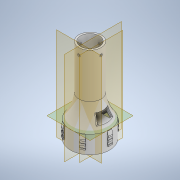
# Autodesk Inventor part: Tube_1
Saved by Autodesk Inventor 2022.3 (Build 263350000, 350)
## iProperties
Created: 2023-03-28
Part Number: Tube_1
Material: Generic
Document SubType Name: Modeling
Designer: Manuel Hueso Béjar
Density: 1 g/cm^3
Appearance: Default
Author: Manuel Hueso Béjar
Autodesk Inventor part; units mm, degrees
ref_plane "XZ Plane" through (0, 0, 0) normal (0, 1, 0) x (-1, 0, 0)
sketch "Sketch1" plane through (0, 0, 0) normal (0, 1, 0) x (-1, 0, 0)
  circle A0 centre (0, 0) radius 40
  circle A1 centre (0, 0) radius 44
  dimension "d0" = 80
  dimension "d1" = 4
  constraints: 2 centre point, 1 coincident
  measures "d0" diameter of A0
  measures "d1" radial gap between concentric circles of A0 A1
extrude "Extrusion1" add sketch "Sketch1" along normal blind 40
sketch "Sketch2" plane through (0, 0, 0) normal (0, 0, 1) x (1, 0, 0)
  line L0 (44, 40) -> (-44, 40) projected
  line L1 (-44, 40) -> (44, 40)
  line L2 (44, 40) -> (44, 90)
  line L3 (44, 90) -> (-44, 90)
  line L4 (-44, 90) -> (-44, 40)
  line L5 (25, 40) -> (-25, 40)
  arc A0 (-44, 40) -> (-25, 90) centre (-124.5733, 99.2279) ccw
  line L6 (-25, 90) -> (0, 90)
  line L7 (0, 90) -> (0, 190)
  line L8 (0, 190) -> (-25, 190)
  line L9 (-25, 190) -> (-25, 90)
  line L10 (0, 90) -> (0, 40)
  line L11 (0, 40) -> (-44, 40)
  line L12 (-25, 190) -> (-21, 190)
  line L13 (-21, 190) -> (-21, 90)
  line L14 (-21, 90) -> (-25, 90)
  line L15 (-25, 90) -> (-25, 190)
  line L16 (-40, 40) -> (40, 40) projected
  arc A1 (-40, 40) -> (-21, 90) centre (-120.5733, 99.2279) ccw
  line L17 (-21, 90) -> (-41, 90)
  line L18 (-41, 90) -> (-41, 70)
  line L19 (-41, 70) -> (-21, 70)
  line L20 (-21, 70) -> (-21, 90)
  line L21 (-44, 40) -> (-29, 40)
  line L22 (-29, 40) -> (-29, 50)
  line L23 (-29, 50) -> (-44, 50)
  line L24 (-44, 50) -> (-44, 40)
  arc A2 (-40.8057, 40.5923) -> (-21.9957, 90.0923) centre (-120.5733, 99.2279) ccw
  line L25 (-24.94, 70) -> (-29.94, 70)
  line L26 (-29.94, 70) -> (-29.94, 68)
  line L27 (-29.94, 68) -> (-24.94, 68)
  line L28 (-24.94, 68) -> (-24.94, 70)
  line L29 (-37.5296, 50) -> (-32.5296, 50)
  line L30 (-32.5296, 50) -> (-32.5296, 51)
  line L31 (-32.5296, 51) -> (-37.5296, 51)
  line L32 (-37.5296, 51) -> (-37.5296, 50)
  point P0 (0, 0)
  point P1 (0, 90)
  point P2 (-25, 90)
  point P3 (-28.94, 70)
  point P4 (-37.5296, 50)
  point P5 (-33.5296, 50)
  point P6 (-25.9862, 70)
  point P7 (-34.6803, 50)
  point P8 (-25.5743, 68)
  point P9 (-26.6275, 68)
  dimension "d4" = 88
  dimension "d5" = 50
  dimension "d8" = 100
  dimension "d9" = 25
  dimension "d10" = 100
  dimension "d11" = 4
  dimension "d12" = 100
  dimension "d79" = 0
  dimension "d196" = 20
  dimension "d197" = 20
  dimension "d198" = 15
  dimension "d199" = 10
  dimension "d205" = 1
  dimension "d206" = 5
  dimension "d207" = 2
  dimension "d208" = 5
  dimension "d209" = 1
  constraints: 62 end point, 14 parallel, 8 perpendicular, 8 point on circle, 7 horizontal, 3 centre point, 3 point on line, 2 midpoint
  measures "d4" distance of L3.end L2.end
  measures "d5" distance of L2.end L1.end
  measures "d8" radius of A0
  measures "d9" distance of L8.end L7.end
  measures "d10" distance of L7.end L6.end
  measures "d11" distance of L13.end L14.end
  measures "d12" radius of A1
  measures "d79" distance between parallel lines of L3 L6
  measures "d196" distance of L19.end L18.end
  measures "d197" distance of L18.end L17.end
  measures "d198" distance of L23.end L22.end
  measures "d199" distance of L22.end L21.end
  measures "d205" radial gap between concentric circles of A1 A2
  measures "d206" distance of L27.end L26.end
  measures "d207" distance of L26.end L25.end
  measures "d208" distance of L31.end L30.end
  measures "d209" distance of L30.end L29.end
revolve "Revolution1" add sketch "Sketch2" angle 360 about axis through (0, 90, 0) along (0, 1, 0) contours A1 L19 A2 L3 | L3 L9 L8 L13 | A2 L19 A0 L3 | A1 L27 A2 L19 | A2 L27 A0 L19 | A1 L31 A2 L27 | L0 A0 L23 A1 | A2 L31 A0 L27 | A1 L23 A2 L31 | A2 L23 A0 L31
ref_plane "Work Plane1" through (0, 45, 0) normal (0, -1, 0) x (1, 0, 0)
sketch "Sketch3" plane through (0, 45, 0) normal (0, -1, 0) x (1, 0, 0)
  line L0 (-2.5, -37.5) -> (2.5, -37.5)
  line L1 (2.5, -37.5) -> (2.5, 37.5)
  line L2 (2.5, 37.5) -> (-2.5, 37.5)
  line L3 (-2.5, 37.5) -> (-2.5, -37.5)
  circle A0 centre (0, 0) radius 44 projected
  line L4 (-2.5, -37.5) -> (2.5, 37.5) construction
  line L5 (2.5, -37.5) -> (-2.5, 37.5) construction
  line L6 (-37.5, -2.5) -> (37.5, -2.5)
  line L7 (37.5, -2.5) -> (37.5, 2.5)
  line L8 (37.5, 2.5) -> (-37.5, 2.5)
  line L9 (-37.5, 2.5) -> (-37.5, -2.5)
  line L10 (-37.5, -2.5) -> (37.5, 2.5) construction
  line L11 (37.5, -2.5) -> (-37.5, 2.5) construction
  circle A1 centre (0, 0) radius 7.5
  circle A2 centre (0, 0) radius 2.6
  circle A3 centre (0, 0) radius 6.6
  line L12 (37.5, 2.5) -> (2.5, 2.5)
  line L13 (2.5, 2.5) -> (2.5, 12.5)
  line L14 (2.5, 12.5) -> (37.5, 12.5)
  line L15 (37.5, 12.5) -> (37.5, 2.5)
  line L16 (-37.5, 2.5) -> (-2.5, 2.5)
  line L17 (-2.5, 2.5) -> (-2.5, 12.5)
  line L18 (-2.5, 12.5) -> (-37.5, 12.5)
  line L19 (-37.5, 12.5) -> (-37.5, 2.5)
  line L20 (37.5, -2.5) -> (-37.5, -2.5)
  line L21 (-37.5, -2.5) -> (-37.5, -12.5)
  line L22 (-37.5, -12.5) -> (37.5, -12.5)
  line L23 (37.5, -12.5) -> (37.5, -2.5)
  line L24 (-2.5, 37.5) -> (-12.5, 37.5)
  line L25 (-12.5, 37.5) -> (-12.5, -37.5)
  line L26 (-12.5, -37.5) -> (-2.5, -37.5)
  line L27 (-2.5, -37.5) -> (-2.5, 37.5)
  line L28 (2.5, 37.5) -> (12.5, 37.5)
  line L29 (12.5, 37.5) -> (12.5, -37.5)
  line L30 (12.5, -37.5) -> (2.5, -37.5)
  line L31 (2.5, -37.5) -> (2.5, 37.5)
  point P0 (7.0711, 2.5)
  point P1 (2.5, 7.0711)
  point P2 (-2.5, 7.0711)
  point P3 (-7.0711, 2.5)
  point P4 (-7.0711, -2.5)
  point P5 (-2.5, -7.0711)
  point P6 (2.5, -7.0711)
  point P7 (7.0711, -2.5)
  point P8 (2.5, 0.7141)
  point P9 (2.5, -0.7141)
  point P10 (12.5, 12.5)
  point P11 (-2.5, -0.7141)
  point P12 (-2.5, 0.7141)
  point P13 (-12.5, 12.5)
  point P14 (0.7141, -2.5)
  point P15 (-0.7141, -2.5)
  point P16 (-12.5, -12.5)
  point P17 (-2.5, -37.5)
  point P18 (12.5, -12.5)
  dimension "d15" = 5
  dimension "d16" = 75
  dimension "d17" = 75
  dimension "d18" = 5
  dimension "d19" = 15
  dimension "d20" = 5.2
  dimension "d165" = 4
  dimension "d181" = 10
  dimension "d182" = 10
  dimension "d202" = 10
  dimension "d203" = 10
  dimension "d204" = 10
  constraints: 64 end point, 14 parallel, 7 horizontal, 7 perpendicular, 4 midpoint, 3 centre point, 2 coincident, 2 point on line
  measures "d15" distance of L2.end L1.end
  measures "d16" distance of L1.end L0.end
  measures "d17" distance of L8.end L7.end
  measures "d18" distance of L7.end L6.end
  measures "d19" diameter of A1
  measures "d20" diameter of A2
  measures "d165" radial gap between concentric circles of A2 A3
  measures "d181" distance of L12.end L13.end
  measures "d182" distance of L17.end L16.end
  measures "d202" distance of L21.end L20.end
  measures "d203" distance of L26.end L25.end
  measures "d204" distance of L29.end L30.end
extrude "Extrusion2" add sketch "Sketch3" against normal blind 5 contours L3 L22 L1 L0 | L26 L25 L22 L3 | L1 L22 L29 L30 | L22 L25 L6 A1 L3 | L3 A1 L1 L22 | L1 A1 L6 L29 L22 | A1 L6 A3 L3 | L3 A3 L1 A1 | L22 L21 L6 L25 | L1 A3 L6 A1 | L29 L6 L23 L22 | A3 L6 L3 | L3 L6 A2 L1 A3 | A1 L8 A3 L6 | L6 L25 L8 A1 | L6 L9 L8 L25 | L1 L6 A3 | A1 L8 L29 L6 | L6 A3 L8 A1 | L29 L8 L7 L6 | L6 A3 L8 L3 A2 | L3 A2 L6 | A1 L3 A3 L8 | L8 L25 L18 L3 A1 | L8 L19 L18 L25 | L6 A2 L1 | L1 A2 L8 A3 L6 | L29 L14 L15 L8 | L8 A1 L1 L14 L29 | A2 L3 | L6 A2 | A3 L3 L8 | A1 L1 A3 L3 | L3 L2 L1 A1 | L25 L24 L3 L18 | L1 A2 | L8 A3 L1 A1 | L14 L1 L28 L29 | L3 L8 A2 | L3 A3 L1 L8 A2 | A2 L8 L1 | L8 L1 A3
sketch "Sketch18" plane through (0, 0, 0) normal (0, -1, 0) x (1, 0, 0)
  line L0 (-42, 5) -> (-46, 5)
  line L1 (-46, 5) -> (-46, -5)
  line L2 (-46, -5) -> (-42, -5)
  line L3 (-42, -5) -> (-42, 5)
  circle A0 centre (0, 0) radius 44 projected
  line L4 (-42, 5) -> (-46, -5) construction
  line L5 (-46, 5) -> (-42, -5) construction
  circle A1 centre (0, 0) radius 44
  point P0 (-44, 0)
  point P1 (-43.715, -5)
  point P2 (-43.715, 5)
  dimension "d106" = 4
  dimension "d107" = 10
  constraints: 12 end point, 2 midpoint, 2 parallel, 1 coincident, 1 horizontal, 1 horizontal alignment, 1 perpendicular, 4 other
  measures "d106" distance of L2.end L1.end
  measures "d107" distance of L1.end L0.end
extrude "Extrusion11" add sketch "Sketch18" against normal blind 30 contours A0 L2 L1 L0
sketch "Sketch19" plane through (-43.715, 0, -5) normal (0, 0, -1) x (-1, 0, 0)
  line L0 (0, 30) -> (2.285, 30) projected
  line L1 (0, 30) -> (2.285, 30)
  line L2 (2.285, 30) -> (2.285, 40)
  line L3 (2.285, 40) -> (0, 40)
  line L4 (0, 40) -> (0, 30)
  line L5 (0, 40) -> (2.285, 30)
  point P0 (-43.715, 0)
  dimension "d110" = 10
  constraints: 10 end point, 2 parallel, 1 horizontal, 1 perpendicular
  measures "d110" distance of L2.end L1.end
extrude "Extrusion12" add sketch "Sketch19" against normal up to surface (10 mm away) contours L4 L5 L0
extrude "Extrusion13" cut sketch "Sketch18" against normal blind 10 contours A0 L2 L1 L0
pattern_circular "Circular Pattern2" count 6 over 360 about axis through (0, 0, 0) along (0, 1, 0) of "Extrusion11", "Extrusion12", "Extrusion13"
sketch "Sketch20" plane through (0, 0, 0) normal (0, 0, 1) x (1, 0, 0)
  line L0 (-46, 0) -> (-43.715, 0) projected
  line L1 (-46, 0) -> (-45, 0)
  line L2 (-45, 0) -> (-45, 10)
  line L3 (-45, 10) -> (-46, 10)
  line L4 (-46, 10) -> (-46, 0)
  line L5 (-46, 10) -> (-45, 10)
  line L6 (-45, 10) -> (-45, 13)
  line L7 (-45, 13) -> (-46, 13)
  line L8 (-46, 13) -> (-46, 10)
  line L9 (-46, 13) -> (-45, 13)
  line L10 (-45, 13) -> (-45, 18)
  line L11 (-45, 18) -> (-46, 18)
  line L12 (-46, 18) -> (-46, 13)
  line L13 (-46, 18) -> (-45, 18)
  line L14 (-45, 18) -> (-45, 22)
  line L15 (-45, 22) -> (-46, 22)
  line L16 (-46, 22) -> (-46, 18)
  line L17 (-46, 22) -> (-45, 22)
  line L18 (-45, 22) -> (-45, 27)
  line L19 (-45, 27) -> (-46, 27)
  line L20 (-46, 27) -> (-46, 22)
  line L21 (0, 0) -> (0, 10)
  line L22 (0, 0) -> (10, 0) construction
  line L23 (-46, 16) -> (-46, 22)
  line L24 (-46, 7) -> (-46, 13)
  line L25 (-46, 27) -> (-45, 27)
  line L26 (-45, 27) -> (-45, 30)
  line L27 (-45, 30) -> (-46, 30)
  line L28 (-46, 30) -> (-46, 27)
  line L29 (-45, 22) -> (-47, 22)
  line L30 (-47, 22) -> (-47, 27)
  line L31 (-47, 27) -> (-45, 27)
  line L32 (-45, 27) -> (-45, 22)
  line L33 (-45, 13) -> (-47, 13)
  line L34 (-47, 13) -> (-47, 18)
  line L35 (-47, 18) -> (-45, 18)
  line L36 (-45, 18) -> (-45, 13)
  dimension "d113" = 1
  dimension "d114" = 10
  dimension "d115" = 1
  dimension "d116" = 3
  dimension "d117" = 1
  dimension "d118" = 5
  dimension "d119" = 1
  dimension "d120" = 4
  dimension "d121" = 1
  dimension "d122" = 5
  dimension "d123" = 10
  dimension "d124" = 90
  dimension "d133" = 1
  dimension "d134" = 3
  dimension "d138" = 2
  dimension "d139" = 5
  dimension "d140" = 2
  dimension "d141" = 5
  constraints: 72 end point, 16 parallel, 9 horizontal, 9 perpendicular, 1 vertical
  measures "d113" distance of L3.end L2.end
  measures "d114" distance of L2.end L1.end
  measures "d115" distance of L7.end L6.end
  measures "d116" distance of L6.end L5.end
  measures "d117" distance of L11.end L10.end
  measures "d118" distance of L10.end L9.end
  measures "d119" distance of L15.end L14.end
  measures "d120" distance of L14.end L13.end
  measures "d121" distance of L19.end L18.end
  measures "d122" distance of L18.end L17.end
  measures "d123" distance of L21.start L21.end
  measures "d124" angle of L22 L21
  measures "d133" distance of L27.end L26.end
  measures "d134" distance of L26.end L25.end
  measures "d138" distance of L30.end L31.end
  measures "d139" distance of L29.end L30.end
  measures "d140" distance of L34.end L35.end
  measures "d141" distance of L33.end L34.end
revolve "Revolution4" cut sketch "Sketch20" angle 360 about axis through (0, 0, 0) along (0, 1, 0) contours L7 L12 L11 L10 | L33 L34 L35 L12 | L15 L20 L19 L18 | L29 L30 L31 L20
ref_plane "Work Plane3" through (25, 0, 0) normal (1, 0, 0) x (0, 1, 0)
ref_plane "Work Plane4" through (0, 0, 25) normal (0, 0, 1) x (1, 0, 0)
sketch "Sketch21" plane through (0, 0, 25) normal (0, 0, 1) x (1, 0, 0)
  line L0 (21, 190) -> (-21, 190) projected
  line L1 (0, 190) -> (0, 160)
  line L2 (0, 175) -> (25, 175)
  line L3 (25, 90) -> (25, 190) projected
  point P0 (0, 0)
  dimension "d145" = 30
  constraints: 4 end point, 2 midpoint, 1 horizontal, 1 point on line, 1 vertical
  measures "d145" distance of L1.start L1.end
hole "Hole5" at (0, 175, 25) direction (0, 0, -1) diameter 3.4 depth 4.2 countersink diameter 5.9 countersink angle 90
sketch "Sketch22" plane through (25, 0, 0) normal (1, 0, 0) x (0, 1, 0)
  line L0 (190, -21) -> (190, 21) projected
  line L1 (190, 0) -> (160, 0)
  line L2 (190, 0) -> (220, 0) construction
  line L3 (175, 0) -> (175, -25)
  line L4 (90, -25) -> (190, -25) projected
  point P0 (0, 0)
  dimension "d153" = 30
  dimension "d154" = 180
  constraints: 6 end point, 2 horizontal, 2 midpoint, 1 collinear, 1 point on line, 1 vertical
  measures "d153" distance of L1.start L1.end
  measures "d154" angle of L1 L2
hole "Hole6" at (25, 175, 0) direction (-1, 0, 0) diameter 3.4 depth 4.2 countersink diameter 5.9 countersink angle 90
mirror "Mirror1" about plane through (0, 0, 0) normal (0, 0, 1) of "Hole5"
mirror "Mirror2" about plane through (0, 0, 0) normal (1, 0, 0) of "Hole6"
extrude "Extrusion15" add sketch "Sketch3" against normal blind 10 contours A3 L6 L3 | L3 L6 A2 L1 A3 | L1 L6 A3 | L6 A3 L8 L3 A2 | L3 A2 L6 | L6 A2 L1 | L1 A2 L8 A3 L6 | A3 L3 L8 | L3 L8 A2 | L3 A3 L1 L8 A2 | A2 L8 L1 | L8 L1 A3
ref_plane "Work Plane5" through (6.6, 0, 0) normal (1, 0, 0) x (0, 1, 0)
sketch "Sketch24" plane through (6.6, 0, 0) normal (1, 0, 0) x (0, 1, 0)
  line L0 (55, 2.6) -> (55, -2.6) projected
  line L1 (55, 0) -> (50, 0)
  line L2 (50, 12.5) -> (50, -2.5) projected
  line L3 (52.5, 0) -> (52.5, -2)
  point P0 (0, 0)
  point P1 (50, -12.5)
  point P2 (50, 31.1124)
  dimension "d184" = 5
  dimension "d185" = 2
  constraints: 4 end point, 2 midpoint, 1 point on line, 1 vertical
  measures "d184" distance of L1.start L1.end
  measures "d185" distance of L3.start L3.end
revolve "Revolution5" cut sketch "Sketch2" angle 210 about axis through (0, 90, 0) along (0, -1, 0) contours A1 L27 A2 L19 | A2 L27 A0 L19 | A1 L31 A2 L27 | A2 L31 A0 L27 | A1 L23 A2 L31 | A2 L23 A0 L31
revolve "Revolution6" add sketch "Sketch2" angle 150 about axis through (0, 90, 0) along (0, -1, 0) contours A1 L19 A2 L3 | A2 L19 A0 L3 | A1 L27 A2 L19 | A2 L27 A0 L19 | A1 L31 A2 L27 | L0 A0 L23 A1 | A2 L31 A0 L27 | A1 L23 A2 L31 | A2 L23 A0 L31
revolve "Revolution7" cut sketch "Sketch2" angle 360 about axis through (0, 90, 0) along (0, -1, 0) contours A0 L19 L18 L3 | L18 L19 L26 L27 A0 L31 L32 L23 L4 L3 | A0 L27 L26 L19 | L4 L23 A0 | L32 L31 A0
hole "Hole8" at (6.6, 52.5, 0) direction (-1, 0, 0) diameter 2.2 depth 5 counterbore diameter 3.1 counterbore depth 4.1
pattern_circular "Circular Pattern4" count 2 over 90 about axis through (0, 45, 0) along (0, 1, 0) of "Hole8"
revolve "Revolution8" cut sketch "Sketch2" angle 120 about axis through (0, 90, 0) along (0, -1, 0) contours A1 L27 A2 L19 | A2 L27 A0 L19 | A1 L31 A2 L27 | A2 L31 A0 L27 | A1 L23 A2 L31 | A2 L23 A0 L31
revolve "Revolution9" add sketch "Sketch2" angle 60 about axis through (0, 90, 0) along (0, -1, 0) contours A1 L27 A2 L19 | A2 L27 A0 L19 | A1 L31 A2 L27 | A2 L31 A0 L27 | A1 L23 A2 L31 | A2 L23 A0 L31
revolve "Revolution10" add sketch "Sketch2" angle 210 about axis through (0, 90, 0) along (0, -1, 0) contours A1 L27 A2 L19 | A1 L31 A2 L27 | A1 L23 A2 L31
revolve "Revolution11" cut sketch "Sketch2" angle 205 about axis through (0, 90, 0) along (0, -1, 0) contours A1 L31 A2 L27 | A1 L23 A2 L31
revolve "Revolution12" add sketch "Sketch2" angle 155 about axis through (0, 90, 0) along (0, -1, 0) contours A1 L31 A2 L27 | A1 L23 A2 L31
revolve "Revolution13" cut sketch "Sketch2" angle 115 about axis through (0, 90, 0) along (0, -1, 0) contours A1 L31 A2 L27 | A1 L23 A2 L31
revolve "Revolution14" add sketch "Sketch2" angle 65 about axis through (0, 90, 0) along (0, -1, 0) contours A1 L31 A2 L27 | A1 L23 A2 L31
body "Solid1"
